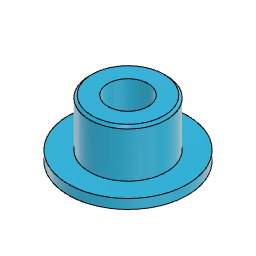
Rondelle-rotation_arbre_croix_de_malte_KOSMOS3-0 (Autodesk Fusion 360 design; units mm, degrees)
Autodesk Fusion 360 part; units mm, degrees
sketch "Esquisse1" plane through (0, 0, 0) normal (0, 0, 1) x (1, 0, 0)
  circle A0 centre (0, 0) radius 8.05
  circle A1 centre (0, 0) radius 4.2
  dimension "d1" = 16.1
  dimension "d2" = 8.4
  constraint coincident A0.centre A1.centre
  constraint concentric A0 A1
  measures "d1" diameter of A0
  measures "d2" diameter of A1
extrude "Extrusion1" add sketch "Esquisse1" along normal blind 10
sketch "Esquisse2" plane through (0, 0, 0) normal (0, 0, -1) x (1, 0, 0)
  circle A0 centre (0, 0) radius 4.2
  circle A1 centre (0, 0) radius 8.05
  circle A2 centre (0, 0) radius 12.5
  dimension "d5" = 25
  constraint concentric A0 A2
  measures "d5" diameter of A2
extrude "Extrusion2" add sketch "Esquisse2" along normal blind 2 contours A1 | A2
chamfer "Chanfrein1" distance 0.5 angle 45 1 edges at (-7.5052, -2.911, 10)
chamfer "Chanfrein2" distance 0.2 angle 45 1 edges at (-3.9158, -1.5188, -2)
sketch "Esquisse3" plane through (0, 0, -2) normal (0, 0, -1) x (1, 0, 0)
  circle A0 centre (0, 0) radius 12.5
  circle A1 centre (0, 0) radius 4.4
